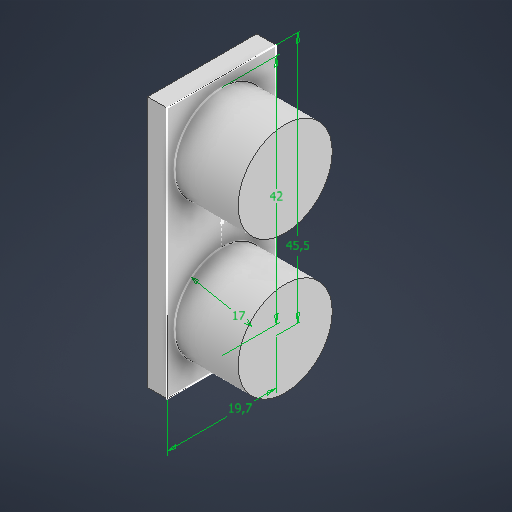
# Autodesk Inventor part: ultrasonic
Saved by Autodesk Inventor 2025.2 (Build 292293000, 293)
## iProperties
Created: 2024-12-17
Part Number: ultrasonic
Material: Generic
Document SubType Name: Modeling
Designer: antem
Density: 1 g/cm^3
Appearance: Default
Author: antem
Autodesk Inventor part; units mm, degrees
ref_plane "YZ Plane" through (0, 0, 0) normal (1, 0, 0) x (0, 1, 0)
ref_plane "XZ Plane" through (0, 0, 0) normal (0, 1, 0) x (-1, 0, 0)
ref_plane "XY Plane" through (0, 0, 0) normal (0, 0, 1) x (1, 0, 0)
sketch "Sketch1" plane through (0, 0, 0) normal (1, 0, 0) x (0, 1, 0)
  line L0 (9.85, 22.75) -> (-9.85, 22.75)
  line L1 (-9.85, 22.75) -> (-9.85, -22.75)
  line L2 (-9.85, -22.75) -> (9.85, -22.75)
  line L3 (9.85, -22.75) -> (9.85, 22.75)
  circle A0 centre (0, 12.5) radius 8.5
  circle A1 centre (0, -12.5) radius 8.5
  line L4 (0, -12.5) -> (0, 12.5) construction
  point P0 (0, 0)
  point P1 (0, 0)
  point P2 (9.85, 0)
  point P3 (0, -22.75)
  dimension "d0" = 45.5
  dimension "d1" = 17
  dimension "d3" = 42
  dimension "d4" = 19.7
  constraints: 10 end point, 3 midpoint, 2 centre point, 2 coincident, 2 parallel, 2 vertical alignment, 1 equal radius, 1 horizontal, 1 horizontal alignment, 1 perpendicular, 1 vertical
  measures "d0" distance of L2.end L0.start
  measures "d1" diameter of A1
  measures "d4" distance of L1.end L2.end
extrude "Extrusion1" add sketch "Sketch1" against normal blind 3.5 contours L3 L2 L1 L0 | A0 | A1
extrude "Extrusion2" add sketch "Sketch1" along normal blind 11.5 contours A0 | A1
body "Solid1"
